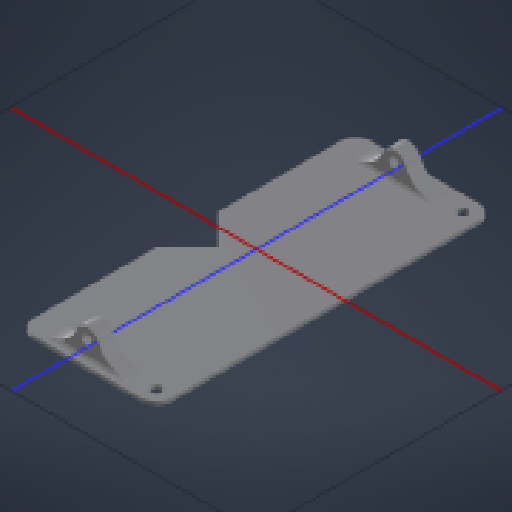
# Autodesk Inventor part: match_loader
Saved by Autodesk Inventor 2025.2 (Build 292293000, 293)
## iProperties
Created: 2025-12-09
Part Number: match_loader
Material: Generic
Document SubType Name: Modeling
Designer: cloudy
Density: 1 g/cm^3
Appearance: Smooth - Dark Gray
Author: cloudy
Autodesk Inventor part; units mm, degrees
ref_plane "YZ Plane" through (0, 0, 0) normal (1, 0, 0) x (0, 1, 0)
ref_plane "XZ Plane" through (0, 0, 0) normal (0, 1, 0) x (-1, 0, 0)
ref_plane "XY Plane" through (0, 0, 0) normal (0, 0, 1) x (1, 0, 0)
sketch "Sketch1" plane through (0, 0, 0) normal (0, 1, 0) x (-1, 0, 0)
  line L0 (28.575, 69.85) -> (-28.575, 69.85)
  line L1 (-28.575, -69.85) -> (28.575, -69.85)
  line L2 (28.575, 69.85) -> (-28.575, -69.85) construction
  line L3 (-28.575, 69.85) -> (28.575, -69.85) construction
  line L4 (0, 0) -> (-53.721, 0) construction
  line L5 (-28.575, 69.85) -> (-28.575, -69.85)
  line L6 (-28.575, -35.3838) -> (-28.575, -69.85)
  line L7 (28.575, 12.7) -> (15.875, 0)
  line L8 (15.875, 0) -> (28.575, -12.7)
  line L9 (28.575, -69.85) -> (28.575, -12.7)
  line L10 (28.575, 12.7) -> (28.575, 69.85)
  point P0 (-12.7, 0)
  point P1 (-28.575, 0)
  dimension "d0" = 57.15
  dimension "d1" = 139.7
  dimension "d4" = 12.7
  dimension "d27" = 90
  dimension "d29" = 12.7
  constraints: 22 end point, 5 parallel, 3 midpoint, 3 perpendicular, 2 horizontal, 2 point on line
  measures "d0" distance of L1.start L1.end
  measures "d1" distance of L1.start L0.end
  measures "d4" distance of L4.start point (-12.7, 0)
  measures "d27" angle of L8 L7
  measures "d29" horizontal distance of L7.start L7.end
extrude "Extrusion1" add sketch "Sketch1" along normal blind 1.5
ref_plane "Work Plane1" through (-28.575, 0, 63.5) normal (0, 0, 1) x (1, 0, 0)
sketch "Sketch2" plane through (-28.575, 0, 63.5) normal (0, 0, 1) x (1, 0, 0)
  circle A0 centre (25.4, 7.85) radius 2.1844
  arc A1 (29.8365, 9.5818) -> (20.9635, 9.5818) centre (25.4, 7.85) ccw
  arc A2 (9.133, 1.5) -> (20.9635, 9.5818) centre (9.133, 14.2) ccw
  arc A3 (29.8365, 9.5818) -> (41.667, 1.5) centre (41.667, 14.2) ccw
  line L0 (0, 1.5) -> (57.15, 1.5) projected
  line L1 (0, 0) -> (0, 1.5) projected
  point P0 (9.133, 1.5)
  dimension "d9" = 4.3688
  dimension "d10" = 9.525
  dimension "d11" = 12.7
  dimension "d12" = 12.7
  dimension "d17" = 6.35
  dimension "d26" = 25.4
  constraints: 6 point on circle, 4 centre point, 4 tangent, 1 coincident, 1 point on line
  measures "d9" diameter of A0
  measures "d10" diameter of A1
  measures "d11" radius of A2
  measures "d12" radius of A3
  measures "d17" distance from line of L0 A0.centre
  measures "d26" distance from line of L1 A0.centre
extrude "Extrusion2" add sketch "Sketch2" along normal mid plane 6.35
chamfer "Chamfer1" distance 0.7937 angle 45 2 edges at (-3.175, 1.5, 66.675) (-3.175, 1.5, 60.325)
fillet "Fillet1" radius 6.35 2 edges at (-28.575, 0.75, 69.85) (28.575, 0.75, 69.85)
mirror "Mirror1" about plane through (0, 0, 0) normal (0, 0, 1) of "Extrusion2", "Chamfer1", "Fillet1"
sketch "Sketch3" plane through (0, 0, 0) normal (0, -1, 0) x (1, 0, 0)
  arc A0 (28.575, 63.5) -> (22.225, 69.85) centre (22.225, 63.5) ccw projected
  circle A1 centre (22.225, 63.5) radius 2.1844
  arc A2 (22.225, -69.85) -> (28.575, -63.5) centre (22.225, -63.5) ccw projected
  circle A3 centre (22.225, -63.5) radius 2.1844
  point P0 (0, 0)
  dimension "d22" = 4.3688
  dimension "d23" = 4.3688
  constraints: 2 centre point, 2 coincident
  measures "d22" diameter of A1
  measures "d23" diameter of A3
extrude "Extrusion3" cut sketch "Sketch3" against normal through all
body "Solid1"
